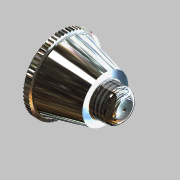
# Autodesk Inventor part: YTP-AP-E07-R1.0
Saved by Autodesk Inventor 2020.4 (Build 244396010, 396A)
## iProperties
RuleStatus: InUse
AfterDocNew0: iPropertyEnforcement
BeforeDocSave0: Materialprüfung
Created: 2021-08-29
Part Number: YTP-AP-E07-R1.0
Material: Allgemein
Document SubType Name: Modeling
Designer: Uwe Wieser
Mass: 0.144522 g
Surface Area: 4.24455 cm^2
Volume: 0.144522 cm^3
Density: 1 g/cm^3
Appearance: Chrom - poliert
Project: Airbrush
Description: Düsenkappe
Werkstoff: 1.4301
Author: Uwe Wieser
Autodesk Inventor part; units mm, degrees
ref_plane "YZ Plane" through (0, 0, 0) normal (1, 0, 0) x (0, 1, 0)
ref_plane "XZ Plane" through (0, 0, 0) normal (0, 1, 0) x (-1, 0, 0)
ref_plane "XY Plane" through (0, 0, 0) normal (0, 0, 1) x (1, 0, 0)
sketch "Skizze1" plane through (0, 0, 0) normal (0, 0, 1) x (1, 0, 0)
  line L0 (-8.5, 4.25) -> (-9, 4.25)
  line L1 (-8.5, 4.75) -> (-8.5, 4.25)
  line L2 (-7.75, 4.75) -> (-9, 4.75)
  line L3 (-2.5, 3) -> (-7.75, 4.25)
  line L4 (-9, 4.25) -> (-9, 3.5)
  line L5 (-5.5, 3.5) -> (-9, 3.5)
  line L6 (-5.5, 3.5) -> (-5.5, 1.75)
  line L7 (-1, 1.75) -> (-5.5, 1.75)
  line L8 (-1, 2) -> (-2.5, 2)
  arc A0 (0, 1) -> (-1, 2) centre (-1, 1) ccw
  arc A1 (-0.25, 1) -> (-1, 1.75) centre (-1, 1) ccw
  line L9 (0, 0.25) -> (0, 1)
  line L10 (0, 0.25) -> (-0.25, 0.25)
  line L11 (-0.25, 1) -> (-0.25, 0.25)
  line L12 (0, -0.95) -> (0, 5.7) projected
  line L13 (-10.8414, 0) -> (2.0485, 0) projected
  line L14 (-2.5, 3) -> (-2.5, 2)
  line L15 (-7.75, 4.75) -> (-7.75, 4.25)
  point P0 (0, 0)
  dimension "d0" = 8.5
  dimension "d1" = 0.5
  dimension "d2" = 7
  dimension "d3" = 3.5
  dimension "d4" = 0.5
  dimension "d5" = 0.25
  dimension "d6" = 1
  dimension "d7" = 0.75
  dimension "d8" = 0.25
  dimension "d9" = 1
  dimension "d10" = 9.5
  dimension "d11" = 9
  dimension "d12" = 3.5
  dimension "d14" = 0.5
  dimension "d15" = 103.392
  dimension "d16" = 8.5
  dimension "d17" = 6
  constraints: 26 end point, 4 point on circle, 2 centre point, 1 parallel, 3 other
  measures "d0" diameter of L0 L13
  measures "d1" distance of L0.start L0.end
  measures "d2" diameter of L5 L13
  measures "d3" diameter of L7 L13
  measures "d4" diameter of L10 L13
  measures "d5" distance of L9.start L10.end
  measures "d6" radius of A0
  measures "d7" radius of A1
  measures "d8" distance between parallel lines of L7 L8
  measures "d9" distance of L3.start L8.end
  measures "d10" diameter of L2 L13
  measures "d11" distance between parallel lines of L12 L4
  measures "d12" distance of L5.start L4.end
  measures "d14" distance of L2.start L3.end
  measures "d15" angle of L15 L3
  measures "d16" diameter of L3.end L13
  measures "d17" diameter of L3.start L13
revolve "Umdrehung1" add sketch "Skizze1" angle 360 about axis through (-10, 0, 0) along (1, 0, 0)
sketch "Skizze2" plane through (-8.5, 0, 0) normal (-1, 0, 0) x (0, 0, 1)
  circle A0 centre (0, 0) radius 4.25 projected
  circle A1 centre (0, 0) radius 4.75 projected
  line L0 (0, -6.65) -> (0, 6.65) projected
  line L1 (-6.65, 0) -> (6.65, 0) projected
  line L2 (-4.6, 0) -> (-4.7476, 0.15)
  circle A2 centre (0, 0) radius 4.75 projected
  line L3 (-4.6, 0) -> (-4.7476, -0.15)
  dimension "d21" = 0.3
  dimension "d22" = 4.6
  constraints: 4 end point, 2 point on circle, 1 point on line, 1 symmetric about line
  measures "d21" distance of L3.end L2.end
  measures "d22" distance from line of L0 L2.start
extrude "Extrusion1" cut sketch "Skizze2" against normal up to surface (0.75 mm away) contours L3 A1 L1 | L1 A1 L2
pattern_circular "Runde Anordnung1" count 65 over 360 about axis through (-10, 0, 0) along (1, 0, 0) of "Extrusion1"
fillet "Rundung1" radius 0.2 3 edges at (-2.5, -2, 0) (-8.5, -4.25, 0) (-7.75, -4.25, 0)
fillet "Rundung2" radius 0.2 1 edges at (-9, -4.25, 0)
thread "Gewinde2" size "M4x0.5" class "6g" standard "ISO Metric profile" full length
thread "Gewinde3" size "M7x0.5" class "6H" standard "ANSI Metric M Profile" length 10
